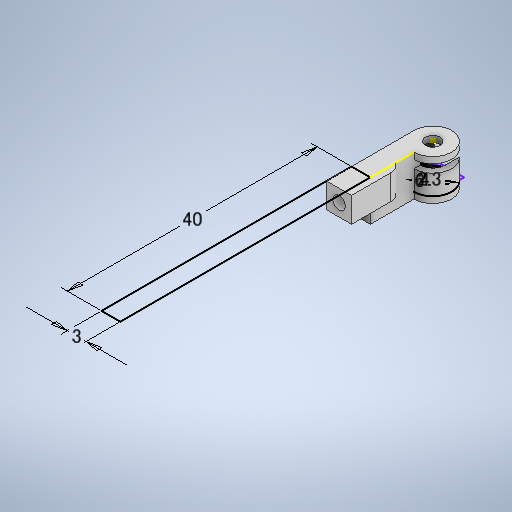
# Autodesk Inventor part: srod1.2
Saved by Autodesk Inventor 2025 (Build 290162000, 162)
## iProperties
Created: 2024-07-27
Part Number: srod1.2
Material: 一般
Document SubType Name: Modeling
Designer: Saigusa
Density: 1 g/cm^3
Appearance: 既定
Author: Saigusa
Autodesk Inventor part; units mm, degrees
ref_plane "YZ Plane" through (0, 0, 0) normal (1, 0, 0) x (0, 1, 0)
ref_plane "XZ Plane" through (0, 0, 0) normal (0, 1, 0) x (-1, 0, 0)
ref_plane "XY Plane" through (0, 0, 0) normal (0, 0, 1) x (1, 0, 0)
sketch "スケッチ1" plane through (0, 0, 0) normal (0, 1, 0) x (-1, 0, 0)
  circle A0 centre (0, 0) radius 1.15
  circle A1 centre (0, 0) radius 2
  circle A2 centre (0, 0) radius 3
  line L0 (0, 0) -> (0, 3)
  line L1 (-2, 0) -> (2, 0)
  line L2 (2, 0) -> (2, -3)
  line L3 (2, -3) -> (-2, -3)
  line L4 (-2, -3) -> (-2, 0)
  line L5 (0, 0) -> (3, 0)
  line L6 (3, 0) -> (3, 3)
  line L7 (3, 3) -> (0, 3)
  line L8 (0, 3) -> (0, 0)
  point P0 (-2, -2.2361)
  point P1 (0, 2)
  point P2 (2, -2.2361)
  dimension "d1" = 4
  dimension "d2" = 6
  dimension "d0" = 2.3
  constraints: 18 end point, 4 parallel, 3 coincident, 2 horizontal, 2 perpendicular, 1 centre point, 1 vertical, 6 other
  measures "d0" diameter of A0
extrude "押し出し1" add sketch "スケッチ1" along normal blind 3.2 contours A1 L4 A2 L0
extrude "押し出し2" add sketch "スケッチ1" along normal blind 4.5 contours L5 A2 L2 | A1 L0 A2 L5 | A2 L7 L6
extrude "押し出し3" add sketch "スケッチ1" against normal blind 1 contours L1 A1 A0 | A0 L0 A1 L1 | A0 L1 A1 L0 | L2 A2 L4 A1 | L5 A2 L2 | A1 L0 A2 L5 | A1 L4 A2 L0 | A2 L7 L6
sketch "スケッチ2" plane through (0, 4.5, 0) normal (0, 1, 0) x (1, 0, 0)
  circle A0 centre (0, 0) radius 1.15
  circle A1 centre (0, 0) radius 2
  circle A2 centre (0, 0) radius 3
  line L0 (0, 0) -> (-3, 0)
  line L1 (-3, 0) -> (-3, -3)
  line L2 (-3, -3) -> (0, -3)
  line L3 (0, -3) -> (0, 0)
  dimension "d9" = 2.3
  dimension "d10" = 4
  dimension "d11" = 6
  constraints: 8 end point, 3 centre point, 3 coincident, 2 parallel, 1 horizontal, 1 perpendicular
  measures "d9" diameter of A0
  measures "d10" diameter of A1
  measures "d11" diameter of A2
extrude "押し出し4" add sketch "スケッチ2" along normal blind 1 contours A0 L0 A1 L3 | A0 L3 A1 L0 | L0 A2 L3 A1 | A1 L3 A2 L0 | A2 L2 L1
sketch "スケッチ3" plane through (-3, -1, 3) normal (0, 0, 1) x (1, 0, 0)
  line L0 (0, 6.5) -> (0, 0) projected
  line L1 (3, 5.5) -> (3, 6.5) projected
  line L2 (0, 0) -> (3, 0)
  line L3 (3, 0) -> (3, 6.5)
  line L4 (3, 6.5) -> (0, 6.5)
  line L5 (0, 6.5) -> (0, 0)
  point P0 (3, 1)
  constraints: 8 end point, 2 parallel, 1 horizontal, 1 perpendicular
extrude "押し出し5" add sketch "スケッチ3" along normal blind 7
sketch "スケッチ4" plane through (-3, -1, 10) normal (0, 0, 1) x (1, 0, 0)
  line L0 (4.15, 0) -> (1.85, 0) projected
  line L1 (3, 0) -> (1.5, 0)
  line L2 (1.5, 0) -> (1.5, 1.5)
  line L3 (1.5, 1.5) -> (3, 1.5)
  line L4 (3, 1.5) -> (3, 0)
  point P0 (3, 1)
  dimension "d16" = 1.5
  dimension "d17" = 1.5
  constraints: 8 end point, 2 parallel, 1 horizontal, 1 midpoint, 1 perpendicular
  measures "d16" distance of L2.end L3.end
  measures "d17" distance of L1.end L2.end
hole "穴1" at (-1.5, 0.5, 10) direction (0, 0, -1) diameter 1 end through all
sketch "スケッチ5" plane through (0, 3.2, 3) normal (1, 0, 0) x (0, 0, -1)
  point P0 (3, -3.2)
sketch "スケッチ7" plane through (0, 5.5, 0) normal (0, 1, 0) x (1, 0, 0)
  line L0 (0, -3) -> (0, -10) projected
  line L1 (0, -10) -> (-3, -10)
  line L2 (-3, -10) -> (-3, -50)
  line L3 (-3, -50) -> (0, -50)
  line L4 (0, -50) -> (0, -10)
  point P0 (0, 0)
  dimension "d33" = 3
  dimension "d34" = 40
  constraints: 8 end point, 2 parallel, 1 horizontal, 1 perpendicular
  measures "d33" distance of L3.end L2.end
  measures "d34" distance of L2.end L1.end
sketch "スケッチ8" plane through (-3, -1, 10) normal (0, 0, 1) x (1, 0, 0)
  line L0 (0, 0) -> (0, 6.5) projected
  line L1 (0, 6.5) -> (4, 6.5)
  line L2 (4, 6.5) -> (4, 2.5)
  line L3 (4, 2.5) -> (0, 2.5)
  line L4 (0, 2.5) -> (0, 6.5)
  point P0 (3, 1)
  dimension "d35" = 4
  dimension "d36" = 4
  constraints: 8 end point, 2 parallel, 1 horizontal, 1 perpendicular
  measures "d35" distance of L2.end L3.end
  measures "d36" distance of L1.end L2.end
extrude "押し出し7" add sketch "スケッチ8" along normal mid plane 8
sketch "スケッチ9" plane through (-3, -1, 14) normal (0, 0, 1) x (1, 0, 0)
  line L0 (0, 0) -> (0, 6.5) projected
  line L1 (0, 6.5) -> (2, 6.5)
  line L2 (2, 6.5) -> (2, 4.5)
  line L3 (2, 4.5) -> (0, 4.5)
  line L4 (0, 4.5) -> (0, 6.5)
  point P0 (3, 1)
  dimension "d39" = 2
  dimension "d40" = 2
  constraints: 8 end point, 2 parallel, 1 horizontal, 1 perpendicular
  measures "d39" distance of L2.end L3.end
  measures "d40" distance of L1.end L2.end
hole "穴2" at (-1, 3.5, 14) direction (0, 0, -1) diameter 2 depth 3 tip angle 118
fillet "フィレット1" radius 2 1 edges at (1, 3.5, 6)
